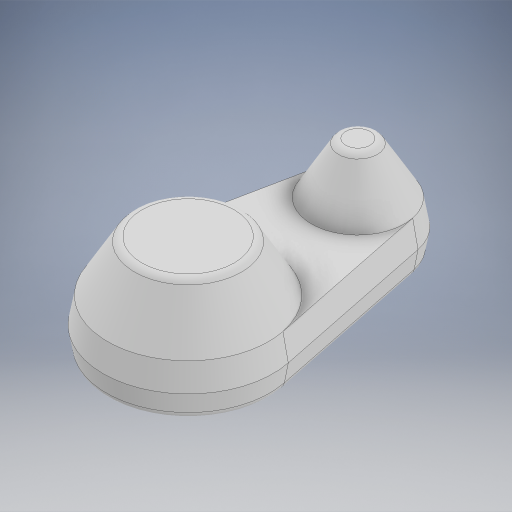
# Autodesk Inventor part: LE-1.1
Saved by Autodesk Inventor 2024 (Build 280153000, 153)
## iProperties
Created: 2024-01-25
Part Number: LE-1.1
Material: Generic
Document SubType Name: Modeling
Designer: Alex
Density: 1 g/cm^3
Appearance: Default
Author: Alex
Autodesk Inventor part; units mm, degrees
ref_plane "YZ Plane" through (0, 0, 0) normal (1, 0, 0) x (0, 1, 0)
ref_plane "XZ Plane" through (0, 0, 0) normal (0, 1, 0) x (-1, 0, 0)
sketch "Sketch1" plane through (0, 0, 0) normal (0, 1, 0) x (-1, 0, 0)
  arc A0 (-48.9898, -10) -> (48.9898, -10) centre (0, 0) ccw construction
  line L0 (0, 0) -> (0, -100) construction
  arc A1 (29.3939, -106) -> (-29.3939, -106) centre (0, -100) ccw construction
  line L1 (48.9898, -10) -> (29.3939, -106)
  line L2 (-48.9898, -10) -> (-29.3939, -106)
  arc A2 (48.9898, -10) -> (-48.9898, -10) centre (0, 0) ccw
  arc A3 (-29.3939, -106) -> (29.3939, -106) centre (0, -100) ccw
  dimension "d0" = 100
  dimension "d1" = 100
  dimension "d2" = 60
  constraints: 8 point on circle, 6 end point, 4 centre point, 4 tangent, 2 coincident, 1 vertical
  measures "d0" diameter of A0
  measures "d1" distance of L0.start L0.end
  measures "d2" diameter of A1
extrude "Extrusion1" add sketch "Sketch1" along normal mid plane 30 draft -10
ref_plane "Work Plane1" through (47.6941, 7.5, -9.7355) normal (0, 1, 0) x (1, 0, 0)
sketch "Sketch2" plane through (0, 15, 0) normal (0, 1, 0) x (1, 0, 0)
  line L0 (-46.3983, 9.471) -> (-26.8024, 105.471) projected
  circle A0 centre (0, 0) radius 47.3551
  constraints: 1 coincident, 3 other
extrude "Extrusion2" add sketch "Sketch2" along normal blind 30 draft -30
sketch "Sketch3" plane through (0, 15, 0) normal (0, 1, 0) x (1, 0, 0)
  arc A0 (26.8024, 105.471) -> (-26.8024, 105.471) centre (0, 100) ccw projected
  circle A1 centre (0, 100) radius 27.3551
  point P0 (0, 0)
  point P1 (-26.8024, 105.471)
  dimension "d7" = 54.7102
  constraints: 1 centre point, 1 coincident
  measures "d7" diameter of A1
extrude "Extrusion3" add sketch "Sketch3" along normal blind 30 draft -30
fillet "Fillet1" radius 5 6 edges at (-30.0346, 45, 0) (-9.8318, 45, -97.9931) (0, -15, -127.3551) (-36.6004, -15, -57.471) (0, -15, 47.3551) (36.6004, -15, -57.471)
body "Solid1"
